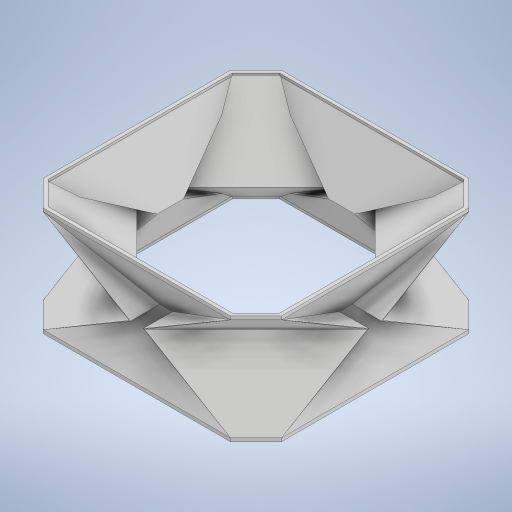
# Autodesk Inventor part: OV-PAM_NEW_SHAPE_5_patterns_1f
Saved by Autodesk Inventor 2024 (Build 280153000, 153)
## iProperties
Created: 2023-06-26
Part Number: OV-PAM_NEW_SHAPE_5_patterns_1f
Material: 일반
Document SubType Name: Modeling
Designer: jsw
Density: 1 g/cm^3
Appearance: 기본값
Author: jsw
Autodesk Inventor part; units mm, degrees
ref_plane "YZ Plane" through (0, 0, 0) normal (1, 0, 0) x (0, 1, 0)
ref_plane "XZ Plane" through (0, 0, 0) normal (0, 1, 0) x (-1, 0, 0)
ref_plane "XY Plane" through (0, 0, 0) normal (0, 0, 1) x (1, 0, 0)
sketch "스케치1" plane through (0, 0, 0) normal (0, 1, 0) x (-1, 0, 0)
  line L0 (28, -11.598) -> (11.598, -28)
  line L1 (11.598, -28) -> (-11.598, -28)
  line L2 (-11.598, -28) -> (-28, -11.598)
  line L3 (-28, -11.598) -> (-28, 11.598)
  line L4 (-28, 11.598) -> (-11.598, 28)
  line L5 (-11.598, 28) -> (11.598, 28)
  line L6 (11.598, 28) -> (28, 11.598)
  line L7 (28, 11.598) -> (28, -11.598)
  line L8 (28, 11.598) -> (28, 22)
  line L9 (11.598, 28) -> (22, 28)
  line L10 (22, 28) -> (28, 22)
  line L11 (-11.598, 28) -> (-22, 28)
  line L12 (-28, 22) -> (-22, 28)
  line L13 (-28, 11.598) -> (-28, 22)
  line L14 (-28, -11.598) -> (-28, -22)
  line L15 (-22, -28) -> (-28, -22)
  line L16 (-11.598, -28) -> (-22, -28)
  line L17 (11.598, -28) -> (22, -28)
  line L18 (28, -22) -> (22, -28)
  line L19 (28, -11.598) -> (28, -22)
  point P0 (0, 0)
  point P1 (0, 0)
  point P2 (0, 0)
  point P3 (28, -11.598)
  point P4 (-28, 11.598)
  point P5 (25, 25)
  point P6 (-25, -25)
  dimension "d7" = 360
  dimension "d28" = 50
  dimension "d29" = 56
  constraints: 40 end point, 2 coincident, 2 horizontal, 2 midpoint, 1 perpendicular, 1 vertical, 46 other
  measures "d28" horizontal distance of point (-25, -25) point (25, 25)
  measures "d29" distance between parallel lines of L5 L1
extrude "돌출1" add sketch "스케치1" along normal blind 12
ref_plane "작업 평면3" through (22, 0, -28) normal (0, -0.5, 0.8660254) x (-1, 0, 0)
ref_plane "작업 평면4" through (28, 0, -22) normal (-0.4545195, -0.7660444, 0.4545195) x (-0.7071068, 0, -0.7071068)
sketch "스케치4" plane through (22, 0, -28) normal (0, 0, -1) x (-1, 0, 0)
  line L0 (0, 0) -> (44, 0) projected
  line L1 (0, 0) -> (20.5, 12)
  line L2 (0, 12) -> (44, 12) projected
  line L3 (50, 0) -> (44, 0) projected
  line L4 (44, 0) -> (23.5, 12)
  point P0 (22, 0)
  point P1 (22, 12)
  dimension "d15" = 1.5
  dimension "d16" = 3
  constraints: 4 end point, 1 midpoint, 1 point on line
  measures "d15" distance of L1.end point (22, 12)
  measures "d16" distance of L1.end L4.end
extrude "돌출2" cut sketch "스케치4" against normal up to surface surface through (22, 0, -28) normal (0, -0.5, 0.8660254)
sketch "스케치5" plane through (28, 0, -22) normal (0.7071068, 0, -0.7071068) x (-0.7071068, 0, -0.7071068)
  line L0 (8.4853, 0) -> (0, 0) projected
  line L1 (0, 0) -> (-20.7846, 12)
  line L2 (0, 12) -> (-31.1127, 12) projected
  line L3 (39.598, 0) -> (8.4853, 0) projected
  line L4 (8.4853, 0) -> (29.2699, 12)
  line L5 (39.598, 12) -> (8.4853, 12) projected
  line L6 (-20.7846, 12) -> (29.2699, 12)
  line L7 (8.4853, 0) -> (0, 0)
  point P0 (4.2426, 0)
  point P1 (0, 12)
  dimension "d19" = 150
  dimension "d20" = 150
  constraints: 8 end point, 2 collinear, 2 point on line
  measures "d19" angle of L4 L0
  measures "d20" angle of L1 L0
extrude "돌출3" cut sketch "스케치5" against normal up to surface surface through (28, 0, -22) normal (-0.4545195, -0.7660444, 0.4545195)
pattern_circular "원형 패턴1" count 4 over 360 about axis through (0, -10, 0) along (0, 1, 0) of "돌출2", "돌출3"
sketch "스케치8" plane through (0, 0, 0) normal (0, -1, 0) x (1, 0, 0)
  line L0 (22, -28) -> (-22, -28) projected
  line L1 (28, -22) -> (22, -28) projected
  line L2 (28, 22) -> (28, -22) projected
  line L3 (22, 28) -> (28, 22) projected
  line L4 (-22, 28) -> (22, 28) projected
  line L5 (-28, 22) -> (-22, 28) projected
  line L6 (-28, -22) -> (-28, 22) projected
  line L7 (-22, -28) -> (-28, -22) projected
  point P0 (0, 0)
extrude "돌출4" add sketch "스케치8" along normal blind 0.8
mirror "미러2" about plane through (0, 12, 0) normal (0, 1, 0) of "돌출2", "돌출3", "원형 패턴1", "돌출4", "돌출1"
shell "쉘2" thickness 0.8 removed faces 2 at (-9.3333, 24.8, 7.3333) at (9.3333, -0.8, -7.3333)
equation "\"d15\" = 0.5 * d16"
